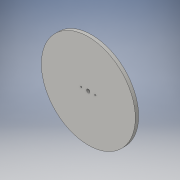
# Autodesk Inventor part: Zoetrope_Board
Saved by Autodesk Inventor 2016 (Build 200138000, 138)
## iProperties
Created: 2019-01-15
Part Number: Zoetrope_Board
Material: Generic
Document SubType Name: Modeling
Designer: student
Density: 1 g/cm^3
Appearance: Default
Author: student
Autodesk Inventor part; units mm, degrees
ref_plane "YZ Plane" through (0, 0, 0) normal (1, 0, 0) x (0, 1, 0)
ref_plane "XZ Plane" through (0, 0, 0) normal (0, 1, 0) x (-1, 0, 0)
ref_plane "XY Plane" through (0, 0, 0) normal (0, 0, 1) x (1, 0, 0)
sketch "Sketch1" plane through (0, 0, 0) normal (0, 0, 1) x (1, 0, 0)
  circle A0 centre (0, 0) radius 63.5
  line L0 (0, 0) -> (9.525, 0) construction
  line L1 (0, 0) -> (-9.525, 0) construction
  circle A1 centre (-9.525, 0) radius 0.9525
  circle A2 centre (9.525, 0) radius 0.9525
  circle A3 centre (0, 0) radius 2.2225
  dimension "d0" = 127
  dimension "d2" = 9.525
  dimension "d3" = 9.525
  dimension "d4" = 1.905
  dimension "d5" = 1.905
  dimension "d6" = 4.445
  constraints: 5 coincident, 4 centre point, 4 end point, 2 horizontal
  measures "d0" diameter of A0
  measures "d2" distance of L0.start L0.end
  measures "d3" distance of L0.start L1.end
  measures "d4" diameter of A1
  measures "d5" diameter of A2
  measures "d6" diameter of A3
extrude "Extrusion1" add sketch "Sketch1" along normal blind 4.572
sketch "Sketch3" plane through (0, 0, 0) normal (0, 0, -1) x (-1, 0, 0)
  point P0 (0, 0)
body "Solid1"
